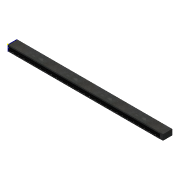
# Autodesk Inventor part: MagneticStrip
Saved by Autodesk Inventor 2016 (Build 200138000, 138)
## iProperties
Created: 2015-05-19
Part Number: MagneticStrip
Material: Steel
Document SubType Name: Modeling
Designer: Andy
Density: 7.85 g/cm^3
Appearance: Plate
Mass: 6649.19 g
Surface Area: 3081.89 cm^2
Volume: 847.03 cm^3
Author: Andy
Autodesk Inventor part; units mm, degrees
ref_plane "YZ Plane" through (0, 0, 0) normal (1, 0, 0) x (0, 1, 0)
ref_plane "XZ Plane" through (0, 0, 0) normal (0, 1, 0) x (-1, 0, 0)
ref_plane "XY Plane" through (0, 0, 0) normal (0, 0, 1) x (1, 0, 0)
sketch "Sketch1" plane through (0, 0, 0) normal (1, 0, 0) x (0, 1, 0)
  line L0 (0, 0) -> (47, 0)
  line L1 (47, 0) -> (47, -30)
  line L2 (47, -30) -> (0, -30)
  line L3 (0, -30) -> (0, 0)
  dimension "d0" = 47
  dimension "d1" = 30
  constraints: 8 end point, 2 parallel, 1 horizontal, 1 perpendicular
  measures "d0" distance of L0.start L0.end
  measures "d1" distance of L0.end L1.end
extrude "Extrusion1" add sketch "Sketch1" along normal blind 794.45
sketch "Sketch2" plane through (0, 0, 0) normal (-1, 0, 0) x (0, 0, 1)
  line L0 (-30, 0) -> (0, 0) projected
  line L1 (0, 0) -> (-12.5, 0)
  line L2 (0, 0) -> (-30, 0) projected
  line L3 (-12.5, 0) -> (-12.5, 37)
  line L4 (-12.5, 37) -> (-19.5, 37)
  line L5 (-19.5, 37) -> (-19.5, 0)
  line L6 (-19.5, 0) -> (-12.5, 0)
  line L7 (-12.5, 0) -> (-7.5, 0)
  line L8 (-12.5, 0) -> (-7.5, 0)
  line L9 (-7.5, 0) -> (-7.5, 37)
  line L10 (-7.5, 37) -> (-24.5, 37)
  line L11 (-24.5, 37) -> (-24.5, 0)
  dimension "d4" = 12.5
  dimension "d5" = 37
  dimension "d6" = 7
  dimension "d9" = 5
  dimension "d10" = 17
  constraints: 20 end point, 3 parallel, 3 perpendicular, 3 point on line, 1 collinear, 1 vertical
  measures "d4" distance of L0.end L1.end
  measures "d5" distance of L1.end L3.end
  measures "d6" distance of L4.end L3.end
  measures "d9" distance of L1.end L7.end
  measures "d10" distance of L9.end L10.end
extrude "Extrusion2" cut sketch "Sketch2" against normal blind 779.45
sketch "Sketch3" plane through (0, 0, 0) normal (0, -1, 0) x (1, 0, 0)
  line L0 (0, -7.5) -> (779.45, -7.5) projected
  line L1 (0, -7.5) -> (23, -7.5)
  line L2 (23, -7.5) -> (23, -12.5)
  line L3 (23, -12.5) -> (0, -12.5)
  line L4 (0, -12.5) -> (0, -7.5)
  line L5 (0, -24.5) -> (779.45, -24.5) projected
  line L6 (0, -24.5) -> (23, -24.5)
  line L7 (23, -24.5) -> (23, -19.5)
  line L8 (23, -19.5) -> (0, -19.5)
  line L9 (0, -19.5) -> (0, -24.5)
  line L10 (28, -7.5) -> (51, -7.5)
  line L11 (51, -7.5) -> (51, -12.5)
  line L12 (51, -12.5) -> (28, -12.5)
  line L13 (28, -12.5) -> (28, -7.5)
  line L14 (28, -24.5) -> (51, -24.5)
  line L15 (51, -24.5) -> (51, -19.5)
  line L16 (51, -19.5) -> (28, -19.5)
  line L17 (28, -19.5) -> (28, -24.5)
  line L18 (56, -7.5) -> (79, -7.5)
  line L19 (79, -7.5) -> (79, -12.5)
  line L20 (79, -12.5) -> (56, -12.5)
  line L21 (56, -12.5) -> (56, -7.5)
  line L22 (56, -24.5) -> (79, -24.5)
  line L23 (79, -24.5) -> (79, -19.5)
  line L24 (79, -19.5) -> (56, -19.5)
  line L25 (56, -19.5) -> (56, -24.5)
  line L26 (84, -7.5) -> (107, -7.5)
  line L27 (107, -7.5) -> (107, -12.5)
  line L28 (107, -12.5) -> (84, -12.5)
  line L29 (84, -12.5) -> (84, -7.5)
  line L30 (84, -24.5) -> (107, -24.5)
  line L31 (107, -24.5) -> (107, -19.5)
  line L32 (107, -19.5) -> (84, -19.5)
  line L33 (84, -19.5) -> (84, -24.5)
  line L34 (112, -7.5) -> (135, -7.5)
  line L35 (135, -7.5) -> (135, -12.5)
  line L36 (135, -12.5) -> (112, -12.5)
  line L37 (112, -12.5) -> (112, -7.5)
  line L38 (112, -24.5) -> (135, -24.5)
  line L39 (135, -24.5) -> (135, -19.5)
  line L40 (135, -19.5) -> (112, -19.5)
  line L41 (112, -19.5) -> (112, -24.5)
  line L42 (140, -7.5) -> (163, -7.5)
  line L43 (163, -7.5) -> (163, -12.5)
  line L44 (163, -12.5) -> (140, -12.5)
  line L45 (140, -12.5) -> (140, -7.5)
  line L46 (140, -24.5) -> (163, -24.5)
  line L47 (163, -24.5) -> (163, -19.5)
  line L48 (163, -19.5) -> (140, -19.5)
  line L49 (140, -19.5) -> (140, -24.5)
  line L50 (163, -7.5) -> (165.5, -7.5)
  line L51 (165.5, -7.5) -> (165.5, 0)
  line L52 (0, 0) -> (794.45, 0) projected
  line L53 (331, -7.5) -> (308, -7.5)
  line L54 (308, -7.5) -> (308, -12.5)
  line L55 (308, -12.5) -> (331, -12.5)
  line L56 (331, -12.5) -> (331, -7.5)
  line L57 (331, -24.5) -> (308, -24.5)
  line L58 (308, -24.5) -> (308, -19.5)
  line L59 (308, -19.5) -> (331, -19.5)
  line L60 (331, -19.5) -> (331, -24.5)
  line L61 (303, -7.5) -> (280, -7.5)
  line L62 (280, -7.5) -> (280, -12.5)
  line L63 (280, -12.5) -> (303, -12.5)
  line L64 (303, -12.5) -> (303, -7.5)
  line L65 (303, -24.5) -> (280, -24.5)
  line L66 (280, -24.5) -> (280, -19.5)
  line L67 (280, -19.5) -> (303, -19.5)
  line L68 (303, -19.5) -> (303, -24.5)
  line L69 (247, -12.5) -> (247, -7.5)
  line L70 (224, -7.5) -> (224, -12.5)
  line L71 (247, -7.5) -> (224, -7.5)
  line L72 (224, -12.5) -> (247, -12.5)
  line L73 (224, -19.5) -> (247, -19.5)
  line L74 (224, -24.5) -> (224, -19.5)
  line L75 (247, -24.5) -> (224, -24.5)
  line L76 (247, -19.5) -> (247, -24.5)
  line L77 (252, -24.5) -> (252, -19.5)
  line L78 (252, -7.5) -> (252, -12.5)
  line L79 (275, -24.5) -> (252, -24.5)
  line L80 (275, -19.5) -> (275, -24.5)
  line L81 (252, -19.5) -> (275, -19.5)
  line L82 (275, -7.5) -> (252, -7.5)
  line L83 (275, -12.5) -> (275, -7.5)
  line L84 (252, -12.5) -> (275, -12.5)
  line L85 (191, -12.5) -> (191, -7.5)
  line L86 (168, -7.5) -> (168, -12.5)
  line L87 (191, -7.5) -> (168, -7.5)
  line L88 (168, -12.5) -> (191, -12.5)
  line L89 (168, -19.5) -> (191, -19.5)
  line L90 (168, -24.5) -> (168, -19.5)
  line L91 (191, -24.5) -> (168, -24.5)
  line L92 (191, -19.5) -> (191, -24.5)
  line L93 (196, -24.5) -> (196, -19.5)
  line L94 (196, -7.5) -> (196, -12.5)
  line L95 (219, -24.5) -> (196, -24.5)
  line L96 (219, -19.5) -> (219, -24.5)
  line L97 (196, -19.5) -> (219, -19.5)
  line L98 (219, -7.5) -> (196, -7.5)
  line L99 (219, -12.5) -> (219, -7.5)
  line L100 (196, -12.5) -> (219, -12.5)
  line L101 (331, -7.5) -> (333.5, -7.5)
  line L102 (667, -7.5) -> (644, -7.5)
  line L103 (644, -7.5) -> (644, -12.5)
  line L104 (644, -12.5) -> (667, -12.5)
  line L105 (667, -12.5) -> (667, -7.5)
  line L106 (667, -24.5) -> (644, -24.5)
  line L107 (644, -24.5) -> (644, -19.5)
  line L108 (644, -19.5) -> (667, -19.5)
  line L109 (667, -19.5) -> (667, -24.5)
  line L110 (639, -7.5) -> (616, -7.5)
  line L111 (616, -7.5) -> (616, -12.5)
  line L112 (616, -12.5) -> (639, -12.5)
  line L113 (639, -12.5) -> (639, -7.5)
  line L114 (639, -24.5) -> (616, -24.5)
  line L115 (616, -24.5) -> (616, -19.5)
  line L116 (616, -19.5) -> (639, -19.5)
  line L117 (639, -19.5) -> (639, -24.5)
  line L118 (583, -12.5) -> (583, -7.5)
  line L119 (560, -7.5) -> (560, -12.5)
  line L120 (583, -7.5) -> (560, -7.5)
  line L121 (560, -12.5) -> (583, -12.5)
  line L122 (560, -19.5) -> (583, -19.5)
  line L123 (560, -24.5) -> (560, -19.5)
  line L124 (583, -24.5) -> (560, -24.5)
  line L125 (583, -19.5) -> (583, -24.5)
  line L126 (588, -24.5) -> (588, -19.5)
  line L127 (588, -7.5) -> (588, -12.5)
  line L128 (611, -24.5) -> (588, -24.5)
  line L129 (611, -19.5) -> (611, -24.5)
  line L130 (588, -19.5) -> (611, -19.5)
  line L131 (611, -7.5) -> (588, -7.5)
  line L132 (611, -12.5) -> (611, -7.5)
  line L133 (588, -12.5) -> (611, -12.5)
  line L134 (527, -12.5) -> (527, -7.5)
  line L135 (504, -7.5) -> (504, -12.5)
  line L136 (527, -7.5) -> (504, -7.5)
  line L137 (504, -12.5) -> (527, -12.5)
  line L138 (504, -19.5) -> (527, -19.5)
  line L139 (504, -24.5) -> (504, -19.5)
  line L140 (527, -24.5) -> (504, -24.5)
  line L141 (527, -19.5) -> (527, -24.5)
  line L142 (532, -24.5) -> (532, -19.5)
  line L143 (532, -7.5) -> (532, -12.5)
  line L144 (555, -24.5) -> (532, -24.5)
  line L145 (555, -19.5) -> (555, -24.5)
  line L146 (532, -19.5) -> (555, -19.5)
  line L147 (555, -7.5) -> (532, -7.5)
  line L148 (555, -12.5) -> (555, -7.5)
  line L149 (532, -12.5) -> (555, -12.5)
  line L150 (504, -7.5) -> (501.5, -7.5)
  line L151 (387, -7.5) -> (387, -12.5)
  line L152 (387, -12.5) -> (364, -12.5)
  line L153 (364, -7.5) -> (387, -7.5)
  line L154 (387, -19.5) -> (364, -19.5)
  line L155 (364, -24.5) -> (387, -24.5)
  line L156 (420, -12.5) -> (420, -7.5)
  line L157 (336, -12.5) -> (336, -7.5)
  line L158 (364, -12.5) -> (364, -7.5)
  line L159 (359, -7.5) -> (359, -12.5)
  line L160 (359, -24.5) -> (359, -19.5)
  line L161 (336, -24.5) -> (359, -24.5)
  line L162 (359, -19.5) -> (336, -19.5)
  line L163 (359, -12.5) -> (336, -12.5)
  line L164 (387, -24.5) -> (387, -19.5)
  line L165 (364, -19.5) -> (364, -24.5)
  line L166 (336, -19.5) -> (336, -24.5)
  line L167 (336, -7.5) -> (359, -7.5)
  line L168 (476, -12.5) -> (476, -7.5)
  line L169 (476, -19.5) -> (476, -24.5)
  line L170 (476, -24.5) -> (499, -24.5)
  line L171 (499, -12.5) -> (476, -12.5)
  line L172 (476, -7.5) -> (499, -7.5)
  line L173 (499, -19.5) -> (476, -19.5)
  line L174 (499, -24.5) -> (499, -19.5)
  line L175 (499, -7.5) -> (499, -12.5)
  line L176 (443, -7.5) -> (443, -12.5)
  line L177 (443, -24.5) -> (443, -19.5)
  line L178 (420, -7.5) -> (443, -7.5)
  line L179 (443, -12.5) -> (420, -12.5)
  line L180 (420, -24.5) -> (443, -24.5)
  line L181 (420, -19.5) -> (420, -24.5)
  line L182 (443, -19.5) -> (420, -19.5)
  line L183 (471, -24.5) -> (471, -19.5)
  line L184 (471, -7.5) -> (471, -12.5)
  line L185 (448, -7.5) -> (471, -7.5)
  line L186 (448, -12.5) -> (448, -7.5)
  line L187 (471, -12.5) -> (448, -12.5)
  line L188 (471, -19.5) -> (448, -19.5)
  line L189 (448, -24.5) -> (471, -24.5)
  line L190 (448, -19.5) -> (448, -24.5)
  line L191 (415, -24.5) -> (415, -19.5)
  line L192 (415, -7.5) -> (415, -12.5)
  line L193 (392, -24.5) -> (415, -24.5)
  line L194 (415, -19.5) -> (392, -19.5)
  line L195 (392, -7.5) -> (415, -7.5)
  line L196 (415, -12.5) -> (392, -12.5)
  line L197 (392, -12.5) -> (392, -7.5)
  line L198 (392, -19.5) -> (392, -24.5)
  line L199 (695, -12.5) -> (695, -7.5)
  line L200 (695, -19.5) -> (695, -24.5)
  line L201 (700, -24.5) -> (700, -19.5)
  line L202 (723, -7.5) -> (700, -7.5)
  line L203 (723, -19.5) -> (723, -24.5)
  line L204 (672, -7.5) -> (672, -12.5)
  line L205 (672, -19.5) -> (695, -19.5)
  line L206 (672, -12.5) -> (695, -12.5)
  line L207 (695, -7.5) -> (672, -7.5)
  line L208 (695, -24.5) -> (672, -24.5)
  line L209 (672, -24.5) -> (672, -19.5)
  line L210 (723, -24.5) -> (700, -24.5)
  line L211 (700, -19.5) -> (723, -19.5)
  line L212 (700, -12.5) -> (723, -12.5)
  line L213 (700, -7.5) -> (700, -12.5)
  line L214 (723, -12.5) -> (723, -7.5)
  line L215 (751, -12.5) -> (751, -7.5)
  line L216 (751, -19.5) -> (751, -24.5)
  line L217 (756, -24.5) -> (756, -19.5)
  line L218 (779, -7.5) -> (756, -7.5)
  line L219 (779, -19.5) -> (779, -24.5)
  line L220 (728, -7.5) -> (728, -12.5)
  line L221 (728, -19.5) -> (751, -19.5)
  line L222 (728, -12.5) -> (751, -12.5)
  line L223 (751, -7.5) -> (728, -7.5)
  line L224 (751, -24.5) -> (728, -24.5)
  line L225 (728, -24.5) -> (728, -19.5)
  line L226 (779, -24.5) -> (756, -24.5)
  line L227 (756, -19.5) -> (779, -19.5)
  line L228 (756, -12.5) -> (779, -12.5)
  line L229 (756, -7.5) -> (756, -12.5)
  line L230 (779, -12.5) -> (779, -7.5)
  dimension "d13" = 23
  dimension "d14" = 5
  dimension "d15" = 5
  dimension "d16" = 23
  dimension "d17" = 5
  dimension "d18" = 5
  dimension "d19" = 23
  dimension "d20" = 5
  dimension "d21" = 5
  dimension "d22" = 23
  dimension "d23" = 5
  dimension "d24" = 5
  dimension "d25" = 23
  dimension "d26" = 5
  dimension "d27" = 5
  dimension "d28" = 23
  dimension "d29" = 5
  dimension "d30" = 5
  dimension "d31" = 2.5
  constraints: 456 end point, 48 symmetric about line, 33 point on line, 24 parallel, 13 perpendicular
  measures "d13" distance of L0.start L1.end
  measures "d14" distance of L1.end L2.end
  measures "d15" distance of L7.end L6.end
  measures "d16" distance of L10.start L10.end
  measures "d17" distance of L10.end L11.end
  measures "d18" distance of L15.end L14.end
  measures "d19" distance of L18.start L19.start
  measures "d20" distance of L19.start L19.end
  measures "d21" distance of L23.end L23.start
  measures "d22" distance of L29.end L27.start
  measures "d23" distance of L27.start L27.end
  measures "d24" distance of L32.start L31.start
  measures "d25" distance of L34.start L35.start
  measures "d26" distance of L35.start L35.end
  measures "d27" distance of L39.end L39.start
  measures "d28" distance of L45.end L43.start
  measures "d29" distance of L43.start L43.end
  measures "d30" distance of L48.start L47.start
  measures "d31" distance of L43.start L50.end
extrude "Extrusion3" add sketch "Sketch3" against normal up to next separate body
sketch "Sketch5" plane through (0, 0, 0) normal (-1, 0, 0) x (0, 0, 1)
  line L0 (0, 0) -> (-7.5, 0) projected
  line L1 (0, 0) -> (-1, 0)
  line L2 (-1, 0) -> (-1, 47)
  line L3 (-1, 47) -> (0, 47)
  line L4 (0, 47) -> (0, 0)
  dimension "d37" = 1
  constraints: 8 end point, 2 parallel, 1 perpendicular, 1 point on line
  measures "d37" distance of L0.start L1.end
extrude "Extrusion4" cut sketch "Sketch5" against normal up to next bodies 1
sketch "Sketch6" plane through (0, 0, 0) normal (-1, 0, 0) x (0, 0, 1)
  line L0 (-30, 47) -> (-31, 47)
  line L1 (-31, 47) -> (-31, 0)
  line L2 (-31, 0) -> (-30, 0)
  line L3 (-30, 0) -> (-30, 47)
  point P0 (0, 0)
  dimension "d40" = 1
  constraints: 8 end point, 2 parallel, 1 horizontal, 1 perpendicular
  measures "d40" distance of L0.start L0.end
extrude "Extrusion5" add sketch "Sketch6" against normal blind 779.45 bodies 1
sketch "Sketch8" plane through (0, 0, 0) normal (-1, 0, 0) x (0, 0, 1)
  line L0 (-1, 0) -> (-1, 47) projected
  line L1 (-31, 47) -> (-31, 0) projected
  line L2 (-31, 0) -> (-24.5, 0) projected
  line L3 (-24.5, 0) -> (-24.5, 37) projected
  line L4 (-24.5, 37) -> (-7.5, 37) projected
  line L5 (-7.5, 37) -> (-7.5, 0) projected
  line L6 (-7.5, 0) -> (-1, 0) projected
  line L7 (-19.5, 0) -> (-19.5, 37) projected
  line L8 (-12.5, 0) -> (-12.5, 37) projected
  line L9 (-1, 0) -> (-1, 47) projected
  line L10 (-1, 47) -> (-31, 47) projected
  line L11 (-31, 47) -> (-31, 0) projected
  line L12 (-31, 0) -> (-24.5, 0) projected
  line L13 (-24.5, 0) -> (-24.5, 37) projected
  line L14 (-24.5, 37) -> (-7.5, 37) projected
  line L15 (-7.5, 37) -> (-7.5, 0) projected
  line L16 (-7.5, 0) -> (-1, 0) projected
  line L17 (-24.5, 0) -> (-24.5, 37)
  line L18 (-24.5, 37) -> (-7.5, 37)
  line L19 (-7.5, 37) -> (-7.5, 0)
  line L20 (-7.5, 37) -> (-7.5, 0) projected
  line L21 (-7.5, 0) -> (-1, 0)
  line L22 (-1, 47) -> (-31, 47)
  line L23 (-1, 0) -> (-1, 47)
  line L24 (-1, 47) -> (-31, 47)
  line L25 (-31, 47) -> (-31, 0)
  line L26 (-31, 0) -> (-24.5, 0)
  line L27 (-1, 0) -> (-30, 0) projected
  line L28 (-24.5, 0) -> (-7.5, 0)
  line L29 (-12.5, 0) -> (-12.5, 37)
  line L30 (-19.5, 0) -> (-19.5, 37)
  line L31 (-24.5, 37) -> (-7.5, 37) projected
  line L32 (-1, 0) -> (-31, 0)
  point P0 (0, 0)
  constraints: 26 end point, 4 perpendicular, 3 horizontal, 3 vertical, 2 collinear, 1 other
body "Solid1"
body "Solid2"
